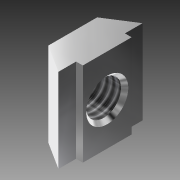
# Autodesk Inventor part: HNTT5-5
Saved by Autodesk Inventor 2015 (Build 190159000, 159)
## iProperties
Category: PARTsolutions
Company: MISUMI
Created: 2014-09-12
Part Number: HNTT5-5
Catalog Web Link: http://us.misumi-ec.com/vona2/detail/110302246150/?HissuCode=HNTT5-5&PNSearch=HNTT5-5
Description: HNTT5-5 - Pre-Assembly Fitting Spring Nuts
Vendor: MISUMI
Document SubType Name: Modeling
Designer: PARTuser1
Manufacturer: MISUMI
Mass: 0.249463 g
Surface Area: 3.33953 cm^2
Volume: 0.249463 cm^3
Density: 1 g/cm^3
Material: Generic
Appearance: PSOLRGB-175-175-175
PSOL_IDENT_0: {\\10.0.0.236\data_v8\23d-libs\misumi\metric\38_al_extrusions_blackets\nuts\hnttss.prj},189 {VTYP=3D
PSOL_IDENT_1: },{NB=HNTT5-5},{LINA=HNTT5-5},{NN=HNTT, HNTTV, HNTTZ, HNTTSN, HNTTSS},{DATE=26.08.2014 02:03:32},{GE
PSOL_IDENT_2: OMDATE=28.12.2010 04:12:00},{VERSION=},{LINEID=20},{LINESUBID=-1},{WBVAR=MAT,M}  {NB=HNTT5-5},{LINA=
PSOL_IDENT_3: HNTT5-5},{KT=DUMMY},{PN=HNTT5-5},{TP=HNTT},{MAT=1010 Steel (or Equivalent)},{ST=Trivalent Chromate},
PSOL_IDENT_4: {NO=5},{M=5},{CFS=HFS5},{CFSW=6},{CFT=20, 40 sq.},{MATT='3','4','5'},{A=5.8},{B=10.0},{D=0.0},{E=3.3
PSOL_IDENT_5: },{T=4.1},{L=10},{MMIN=4.134},{MMAX=5},{TT=6.8},{MATALG='1010 Steel (or Equivalent)','1010 Carbon St
PSOL_IDENT_6: eel Equivalent','V','Thread Locking Adhesive / 1010 Carbon Steel Equivalent','Z','Thread Locking Res
PSOL_IDENT_7: in Coating / 1010 Carbon Steel Equivalent','316 Stainless Steel (or Equivalent)','316 Stainless Stee
PSOL_IDENT_8: l Equivalent, Sintering','303 Stainless Steel','303 Stainless Steel'},{X=0.7},{D11=6}
SUPPLIER: MISUMI
ARTICLENO: HNTT5-5
BOMINFO: HNTT5-5
CREATOR: CADENAS GmbH
Title: HNTT5-5
Author: Cadenas PARTsolutions
Comments: Nuts for Aluminum Extrusions - Pre-Assembly Fitting Spring Nuts, Stainless Plate Type
Autodesk Inventor part; units mm, degrees
sketch "Sketch_4" plane through (0, 0, 0) normal (0, 0, 1) x (1, 0, 0)
  line L0 (-4.1, 2.9) -> (-4.1, -2.9)
  line L1 (-4.1, -2.9) -> (-0.8, -5)
  line L2 (-0.8, -5) -> (-0.8, -2.9)
  line L3 (-0.8, -2.9) -> (0, -2.9)
  line L4 (0, -2.9) -> (0, 2.9)
  line L5 (0, 2.9) -> (-0.8, 2.9)
  line L6 (-0.8, 2.9) -> (-0.8, 5)
  line L7 (-0.8, 5) -> (-4.1, 2.9)
  constraints: 16 end point
extrude "Extrusion1" add sketch "Sketch_4" along normal mid plane 10
sketch "Sketch_5" plane through (0, 0, 0) normal (0, 0, 1) x (1, 0, 0)
  line L0 (0, 0) -> (-4.1, 0)
  line L1 (-4.1, 0) -> (-4.1, 2.5)
  line L2 (-4.1, 2.5) -> (-3.667, 2.067)
  line L3 (-3.667, 2.067) -> (-0.433, 2.067)
  line L4 (-0.433, 2.067) -> (0, 2.5)
  line L5 (0, 2.5) -> (0, 0)
  line L6 (0, 0) -> (-4.1, 0)
  constraints: 14 end point
revolve "Revolution1" cut sketch "Sketch_5" angle 360 about axis through (0, 0, 0) along (1, 0, 0)
thread "Thread1" size "M5x0.8" class "6H" standard "ISO Metric profile" full length
ref_plane "nut_XY" through (0, 0, 0) normal (1, 0, 0) x (0, 0, -1)
ref_plane "nut_YZ" through (0, 0, 0) normal (0, 0, -1) x (0, 1, 0)
ref_plane "nut_ZX" through (0, 0, 0) normal (0, 1, 0) x (1, 0, 0)
ref_plane "to_bolt_XY" through (-4.1, 0, 0) normal (1, 0, 0) x (0, 0, -1)
ref_plane "to_bolt_YZ" through (-4.1, 0, 0) normal (0, 0, -1) x (0, 1, 0)
ref_plane "to_bolt_ZX" through (-4.1, 0, 0) normal (0, 1, 0) x (1, 0, 0)
ref_plane "to_frames_XY" through (-0.8, 0, 0) normal (1, 0, 0) x (0, 0, -1)
ref_plane "to_frames_YZ" through (-0.8, 0, 0) normal (0, 0, -1) x (0, 1, 0)
ref_plane "to_frames_ZX" through (-0.8, 0, 0) normal (0, 1, 0) x (1, 0, 0)
body "Solid1"
